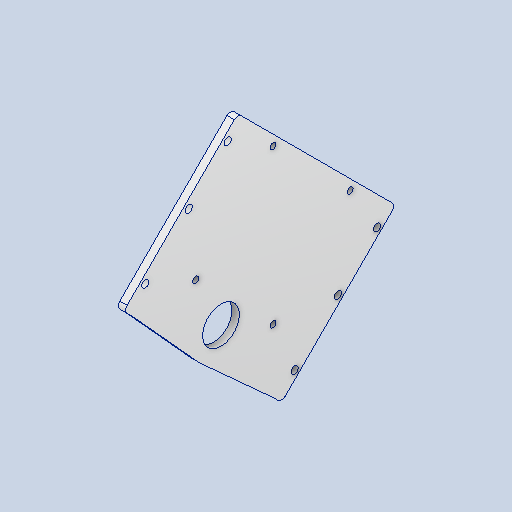
# Autodesk Inventor part: belt_liner_v1_Plate_3
Saved by Autodesk Inventor 2025.1 (Build 291241000, 241)
## iProperties
Created: 2024-12-08
Part Number: belt_liner_v1_Plate_3
Material: アルミニウム 6061
Document SubType Name: Modeling
Designer: haruy
Density: 2.7 g/cm^3
Appearance: アルミニウム - フラット
Author: haruy
Autodesk Inventor part; units mm, degrees
ref_plane "YZ Plane" through (0, 0, 0) normal (1, 0, 0) x (0, 1, 0)
ref_plane "XZ Plane" through (0, 0, 0) normal (0, 1, 0) x (-1, 0, 0)
ref_plane "XY Plane" through (0, 0, 0) normal (0, 0, 1) x (1, 0, 0)
derived "belt_liner_v1_Sketch_Base.ipt"
sketch "スケッチ1" plane through (300, 0, 0) normal (1, 0, 0) x (0, 1, 0)
  circle A0 centre (0, 0) radius 23.875
  circle A1 centre (323.2892, -323.2892) radius 23.875
  line L0 (0, 0) -> (0, -985.832)
  line L1 (14.1421, 50.3106) -> (24.7487, 60.9172)
  line L2 (24.7487, 60.9172) -> (406.5864, -320.9204)
  line L3 (406.5864, -320.9204) -> (395.9798, -331.527)
  line L4 (395.9798, -331.527) -> (14.1421, 50.3106)
  line L5 (0, 0) -> (323.2892, -323.2892)
  line L6 (-50.3106, -14.1421) -> (-60.9172, -24.7487)
  line L7 (-60.9172, -24.7487) -> (289.1006, -374.7666)
  line L8 (289.1006, -374.7666) -> (299.7072, -364.16)
  line L9 (299.7072, -364.16) -> (-50.3106, -14.1421)
  line L10 (22.5524, 63.1136) -> (22.5524, 63.1136)
  line L11 (14.1421, 50.3106) -> (71.3109, -6.8581)
  line L12 (71.3109, -6.8581) -> (67.7754, -10.3937)
  line L13 (67.7754, -10.3937) -> (10.6066, 46.7751)
  line L14 (10.6066, 46.7751) -> (14.1421, 50.3106)
  line L15 (395.9798, -331.527) -> (376.5344, -312.0816)
  line L16 (376.5344, -312.0816) -> (372.9988, -315.6171)
  line L17 (372.9988, -315.6171) -> (392.4443, -335.0625)
  line L18 (392.4443, -335.0625) -> (395.9798, -331.527)
  line L19 (0, -985.832) -> (0, 0)
  circle A2 centre (0, 0) radius 12.5
  circle A3 centre (21.2132, -21.2132) radius 23.5 construction
  circle A4 centre (0, 0) radius 15 construction
  circle A5 centre (21.2132, -21.2132) radius 15 construction
  line L20 (0, 0) -> (0, 0)
  circle A6 centre (-21.2132, 21.2132) radius 15
  circle A7 centre (-21.2132, 21.2132) radius 12.25
  circle A8 centre (0, 0) radius 25.575 construction
  line L21 (0, 0) -> (0, 0)
  line L22 (0, 0) -> (0, 0)
  circle A9 centre (52.7132, -21.2132) radius 1.5
  circle A10 centre (21.2132, -21.2132) radius 31.5 construction
  line L23 (21.2132, -21.2132) -> (49.9041, 7.4777) construction
  circle A11 centre (21.2132, 10.2868) radius 1.5
  circle A12 centre (-10.2868, -21.2132) radius 1.5
  circle A13 centre (21.2132, -52.7132) radius 1.5
  circle A14 centre (21.2132, -52.7132) radius 3
  circle A15 centre (52.7132, -21.2132) radius 3
  circle A16 centre (21.2132, -52.7132) radius 3
  circle A17 centre (-10.2868, -21.2132) radius 3
  circle A18 centre (21.2132, 10.2868) radius 3
  line L24 (23.3345, 12.4081) -> (54.8345, -19.0919) construction
  line L25 (54.8345, -23.3345) -> (23.3345, -54.8345)
  line L26 (19.0919, -54.8345) -> (-12.4081, -23.3345)
  line L27 (-50.3106, -14.1421) -> (-46.7751, -10.6066)
  line L28 (-46.7751, -10.6066) -> (10.3937, -67.7754)
  line L29 (10.3937, -67.7754) -> (6.8581, -71.3109)
  line L30 (6.8581, -71.3109) -> (-50.3106, -14.1421)
  line L31 (-15.7223, 32.1636) -> (22.5579, 12.9685) construction
  line L32 (-32.1636, 15.7223) -> (-12.9685, -22.5579)
  line L33 (84.8528, 0.8132) -> (406.5864, -320.9204)
  line L34 (406.5864, -320.9204) -> (410.4755, -317.0313)
  line L35 (410.4755, -317.0313) -> (88.7419, 4.7023)
  line L36 (88.7419, 4.7023) -> (84.8528, 0.8132)
  circle A19 centre (323.2892, -323.2892) radius 5
  line L37 (299.7072, -364.16) -> (280.9689, -345.4217)
  line L38 (280.9689, -345.4217) -> (284.5044, -341.8861)
  line L39 (284.5044, -341.8861) -> (303.2427, -360.6245)
  line L40 (303.2427, -360.6245) -> (299.7072, -364.16)
  circle A20 centre (319.7537, -319.7537) radius 5
  line L41 (323.2892, -323.2892) -> (417.2615, -417.2615)
  circle A21 centre (337.4314, -337.4314) radius 5
  line L42 (323.2892, -316.2182) -> (340.9669, -333.8958)
  line L43 (316.2182, -323.2892) -> (333.8958, -340.9669)
  circle A22 centre (323.2892, -323.2892) radius 22.175
  circle A23 centre (323.2892, -323.2892) radius 33.875
  line L44 (365.8279, -301.3751) -> (355.2213, -311.9817)
  line L45 (355.2213, -311.9817) -> (358.7568, -315.5172)
  line L46 (358.7568, -315.5172) -> (369.3634, -304.9106)
  line L47 (369.3634, -304.9106) -> (365.8279, -301.3751)
  circle A24 centre (319.7537, -319.7537) radius 10
  circle A25 centre (337.4314, -337.4314) radius 10
  line L48 (326.8248, -312.6826) -> (344.5024, -330.3603)
  line L49 (312.6826, -326.8248) -> (330.3603, -344.5024)
  line L50 (326.8248, -312.6826) -> (318.2892, -304.1471)
  line L51 (312.6826, -312.6826) -> (319.7537, -305.6116)
  line L52 (319.7537, -305.6116) -> (376.5344, -312.0816)
  line L53 (392.4443, -335.0625) -> (303.2427, -360.6245)
  line L54 (344.5024, -330.3603) -> (351.2982, -337.156)
  line L55 (351.2982, -337.156) -> (351.5735, -337.4314)
  line L56 (71.3109, -6.8581) -> (67.7754, -10.3937)
  line L57 (67.7754, -10.3937) -> (90.8632, -33.4815)
  line L58 (90.8632, -33.4815) -> (94.3988, -29.946)
  line L59 (94.3988, -29.946) -> (71.3109, -6.8581)
  line L60 (244.0828, -334.7487) -> (-45.9172, -334.7487)
  line L61 (-45.9172, -334.7487) -> (-45.9172, -349.7487)
  line L62 (-45.9172, -349.7487) -> (244.0828, -349.7487)
  line L63 (244.0828, -349.7487) -> (244.0828, -334.7487)
  line L64 (-60.9172, -24.7487) -> (-60.9172, -604.2835)
  line L65 (-45.9172, -334.7487) -> (-60.9172, -334.7487)
  line L66 (-60.9172, -334.7487) -> (-60.9172, -349.7487)
  line L67 (-60.9172, -349.7487) -> (-45.9172, -349.7487)
  line L68 (-45.9172, -349.7487) -> (-45.9172, -334.7487)
  line L69 (-60.9172, -334.7487) -> (-45.9172, -334.7487)
  line L70 (-45.9172, -334.7487) -> (-45.9172, -44.7487)
  line L71 (-45.9172, -44.7487) -> (-60.9172, -44.7487)
  line L72 (-60.9172, -44.7487) -> (-60.9172, -334.7487)
  line L73 (330.3603, -344.5024) -> (344.5024, -330.3603)
  line L74 (344.5024, -330.3603) -> (351.5735, -337.4314)
  line L75 (351.5735, -337.4314) -> (337.4314, -351.5735)
  line L76 (337.4314, -351.5735) -> (330.3603, -344.5024)
  line L77 (406.5864, -320.9204) -> (395.9798, -331.527)
  line L78 (395.9798, -331.527) -> (399.5153, -335.0625)
  line L79 (399.5153, -335.0625) -> (410.1219, -324.4559)
  line L80 (410.1219, -324.4559) -> (406.5864, -320.9204)
  line L81 (-12.1904, 2.7649) -> (-50.3106, -35.3553)
  line L82 (-12.1904, 2.7649) -> (35.3553, 50.3106)
  line L83 (6.8581, -71.3109) -> (-3.7485, -81.9175)
  line L84 (-22.0264, -35.3553) -> (-36.1685, -49.4975)
  line L85 (-0.8132, -56.5685) -> (-14.9553, -70.7107)
  circle A26 centre (-30.8652, -30.052) radius 1.5
  circle A27 centre (-13.1875, -47.7297) radius 1.5
  circle A28 centre (2.7224, -63.6396) radius 1.5
  line L86 (49.4975, 36.1685) -> (35.3553, 22.0264)
  line L87 (70.7107, 14.9553) -> (56.5685, 0.8132)
  circle A29 centre (30.052, 30.8652) radius 1.5
  circle A30 centre (47.7297, 13.1875) radius 1.5
  circle A31 centre (63.6396, -2.7224) radius 1.5
  line L88 (10.3937, -67.7754) -> (67.7754, -10.3937)
  line L89 (21.2132, 36.1685) -> (-8.4068, 9.2507)
  line L90 (-9.2507, 8.4068) -> (-36.1685, -21.2132)
  circle A32 centre (0, 0) radius 7.5
  line L91 (289.4542, -346.8359) -> (285.9186, -350.3714)
  line L92 (297.9394, -355.3212) -> (294.4039, -358.8567)
  circle A33 centre (287.6864, -348.6036) radius 1.5
  circle A34 centre (296.1717, -357.0889) radius 1.5
  line L93 (381.4841, -317.0313) -> (377.9486, -320.5669)
  line L94 (389.9694, -325.5166) -> (386.4339, -329.0521)
  circle A35 centre (379.7163, -318.7991) radius 1.5
  circle A36 centre (388.2016, -327.2844) radius 1.5
  line L95 (284.5044, -341.8861) -> (312.5571, -312.8104)
  line L96 (312.6826, -326.8248) -> (305.6149, -320.0057)
  circle A37 centre (333.8958, -323.2892) radius 1.25
  circle A38 centre (323.2892, -333.8958) radius 1.25
  line L97 (-45.9172, -64.7487) -> (-60.9172, -64.7487)
  line L98 (-10.3106, -54.1421) -> (-20.9172, -64.7487)
  line L99 (-20.9172, -64.7487) -> (-45.9172, -64.7487)
  line L100 (224.0828, -334.7487) -> (224.0828, -349.7487)
  line L101 (244.0828, -349.7487) -> (264.0828, -349.7487)
  line L102 (264.0828, -349.7487) -> (274.6894, -339.1421)
  line L103 (244.0828, -334.7487) -> (249.0828, -334.7487)
  line L104 (249.0828, -334.7487) -> (259.6894, -324.1421)
  line L105 (-45.9172, -44.7487) -> (-40.9172, -44.7487)
  line L106 (-40.9172, -44.7487) -> (-30.3106, -34.1421)
  line L107 (-45.9172, -329.7487) -> (-60.9172, -329.7487)
  line L108 (-25.9172, -334.7487) -> (-25.9172, -349.7487)
  line L109 (-24.8548, -32.5269) -> (-38.9969, -46.669)
  point P0 (318.2892, -304.1471)
  point P1 (-53.4172, -334.7487)
  point P2 (24.7487, 39.704)
  point P3 (7.6581, 22.6135)
  point P4 (6.6469, 22.9311)
  point P5 (-39.704, -24.7487)
  point P6 (287.6864, -348.6036)
  point P7 (-53.4172, -49.7487)
  point P8 (-53.4172, -59.7487)
  point P9 (-29.451, -45.6084)
  point P10 (-22.3799, -52.6795)
  point P11 (239.0828, -342.2487)
  point P12 (229.0828, -342.2487)
  point P13 (224.0828, -342.2487)
  point P14 (266.1196, -341.179)
  point P15 (259.0486, -334.108)
  point P16 (-45.9172, -342.2487)
  point P17 (-53.4172, -344.7487)
  point P18 (-53.4172, -334.7487)
  point P19 (-40.9172, -342.2487)
  point P20 (-30.9172, -342.2487)
  dimension "d1" = 15
  measures "d1" diameter of A32
extrude "押し出し1" add sketch "スケッチ1" along normal blind 3 contours A0 L5 A2 L82 A18 | A15 | A0 A18 L82 L13 L88 L25 L5 | A18 A0 A11 | A0 A11 A18 | L5 L25 A14 L26 L0 A0 | A0 L0 A2 L5 | L0 L26 A17 A0 | A0 A17 L32 L81 A2 L0 | A2 L0 A32 L5 | L5 A32 L0 A2 L82 | L82 A2 L89 A0 | A0 L89 L82 | A17 A0 A12 | A0 A12 A17 | L26 A14 L88 L28 L0 | L0 L28 L81 A0 L32 A17 L26 | A14 | L82 A2 | L82 L4 L86 L13 | L81 L32 L90 A2 | L28 L29 L9 L0 | L0 L9 L85 L28 | L13 L87 L4 L12 | L86 L4 L87 L13 | L32 A0 A17 | L81 A0 L90 L32 | L32 A0 L81 | L85 L9 L84 L28 | L81 L90 A0 | L84 L9 L109 L28 | L28 L109 L9 L81
fillet "フィレット1" radius 2 4 edges at (301.5, 24.7487, 39.704) (301.5, 71.3109, -6.8581) (301.5, 6.8581, -71.3109) (301.5, -39.704, -24.7487)
sketch "スケッチ2" plane through (303, 6.8581, -68.4825) normal (1, 0, 0) x (0, 0, -1)
  circle A0 centre (-78.7693, 14.3551) radius 1.5 projected
  circle A1 centre (-78.7693, 14.3551) radius 1.5
  circle A2 centre (-78.7693, 14.3551) radius 1.25
  circle A3 centre (-47.2693, -17.1449) radius 1.5 projected
  circle A4 centre (-47.2693, -17.1449) radius 1.5
  circle A5 centre (-47.2693, -17.1449) radius 1.25
  circle A6 centre (-15.7693, 14.3551) radius 1.5 projected
  circle A7 centre (-15.7693, 14.3551) radius 1.5
  circle A8 centre (-15.7693, 14.3551) radius 1.25
  circle A9 centre (-47.2693, 45.8551) radius 1.5 projected
  circle A10 centre (-47.2693, 45.8551) radius 1.25
  circle A11 centre (-47.2693, 45.8551) radius 1.5
  point P0 (-68.4825, -6.8581)
  dimension "d5" = 2.5
  dimension "d6" = 2.5
  dimension "d7" = 2.5
  dimension "d8" = 2.5
  dimension "d9" = 3
  constraints: 8 centre point, 8 coincident
  measures "d5" diameter of A2
  measures "d6" diameter of A5
  measures "d7" diameter of A8
  measures "d8" diameter of A10
  measures "d9" diameter of A11
extrude "押し出し2" add sketch "スケッチ2" against normal up to surface (3 mm away)
thread "ねじ1" size "M2.5x0.45" class "6H" standard "ANSI Metric M Profile" full length
thread "ねじ2" size "M2.5x0.45" class "6H" standard "ANSI Metric M Profile" full length
thread "ねじ3" size "M2.5x0.45" class "6H" standard "ANSI Metric M Profile" full length
thread "ねじ4" size "M2.5x0.45" class "6H" standard "ANSI Metric M Profile" full length
